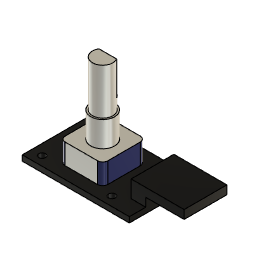
stepper_controller_case v17 (Autodesk Fusion 360 archive; units mm, degrees)
design "UVC_UI_case_KY-040"
Autodesk Fusion 360 part; units mm, degrees
sketch "Sketch1" plane through (0, 0, 0) normal (0, 0, 1) x (1, 0, 0)
  line L0 (4.75, -6.25) -> (-4.75, -6.25)
  line L1 (-6.25, -4.75) -> (-6.25, 4.75)
  line L2 (-4.75, 6.25) -> (4.75, 6.25)
  line L3 (6.25, 4.75) -> (6.25, -4.75)
  line L4 (6.25, -6.25) -> (-6.25, 6.25) construction
  line L5 (-6.25, -6.25) -> (6.25, 6.25) construction
  arc A0 (-4.75, 6.25) -> (-6.25, 4.75) centre (-4.75, 4.75) ccw
  arc A1 (6.25, 4.75) -> (4.75, 6.25) centre (4.75, 4.75) ccw
  arc A2 (4.75, -6.25) -> (6.25, -4.75) centre (4.75, -4.75) ccw
  arc A3 (-6.25, -4.75) -> (-4.75, -6.25) centre (-4.75, -4.75) ccw
  circle A4 centre (0, 0) radius 3.5
  circle A5 centre (0, 0) radius 3
  line L6 (-2.5981, 1.5) -> (2.5981, 1.5)
  line L7 (-6.25, 0) -> (6.25, 0) construction
  line L8 (-13.75, -9.75) -> (17.55, -9.75)
  line L9 (17.55, -9.75) -> (17.55, 9.55)
  line L10 (17.55, 9.55) -> (-13.75, 9.55)
  line L11 (-13.75, 9.55) -> (-13.75, -9.75)
  line L12 (28.75, -4.95) -> (13.25, -4.95)
  line L13 (13.25, -4.95) -> (13.25, 7.55)
  line L14 (13.25, 7.55) -> (28.75, 7.55)
  line L15 (28.75, 7.55) -> (28.75, -4.95)
  circle A6 centre (-10.65, -7.05) radius 1
  circle A7 centre (9.75, -7.05) radius 1
  dimension "d37" = 12.5
  dimension "d38" = 12.5
  dimension "d39" = 1.5
  dimension "d40" = 7
  dimension "d41" = 6
  dimension "d42" = 1.5
  dimension "d43" = 31.3
  dimension "d44" = 19.3
  dimension "d45" = 3.5
  dimension "d46" = 7.5
  dimension "d47" = 15.5
  dimension "d48" = 12.5
  dimension "d49" = 2
  dimension "d50" = 4.3
  dimension "d51" = 2
  dimension "d52" = 3.1
  dimension "d53" = 2.7
  dimension "d54" = 2
  dimension "d55" = 7.8
  dimension "d56" = 2.7
  constraint horizontal L0
  constraint perpendicular L0 L1
  constraint parallel L0 L2
  constraint parallel L1 L3
  constraint coincident L4 A4.centre
  constraint coincident L5 A4.centre
  constraint coincident A4.centre A5.centre
  constraint coincident L4.end L2
  constraint coincident L4.end L1
  constraint tangent L2 A0
  constraint tangent L1 A0
  constraint coincident L5.end L2
  constraint coincident L5.end L3
  constraint tangent L2 A1
  constraint tangent L3 A1
  constraint equal A0 A1
  constraint coincident L4.start L3
  constraint coincident L4.start L0
  constraint tangent L3 A2
  constraint tangent L0 A2
  constraint equal A0 A2
  constraint coincident L5.start L0
  constraint coincident L5.start L1
  constraint tangent L0 A3
  constraint tangent L1 A3
  constraint equal A0 A3
  constraint coincident A5 L6.start
  constraint coincident A5 L6.end
  constraint horizontal L6
  constraint midpoint L1 L7.start
  constraint midpoint L3 L7.end
  constraint horizontal L8
  constraint vertical L9
  constraint horizontal L10
  constraint vertical L11
  constraint horizontal L12
  constraint vertical L13
  constraint horizontal L14
  constraint vertical L15
  measures "d37" distance of L4.end L5.end
  measures "d38" distance of L5.start L4.end
  measures "d39" radius of A0
  measures "d40" diameter of A4
  measures "d41" diameter of A5
  measures "d42" distance of L6 L7
  measures "d43" distance of L8.start L8.end
  measures "d44" distance of L8.start L10.end
  measures "d45" distance of L0 L8
  measures "d46" distance of L1 L11
  measures "d47" distance of L12.start L12.end
  measures "d48" distance of L12.start L14.end
  measures "d49" distance of L10 L14
  measures "d50" distance of L9 L13
  measures "d51" diameter of A6
  measures "d52" distance of L11 A6.centre
  measures "d53" distance of L8 A6.centre
  measures "d54" diameter of A7
  measures "d55" distance of L9 A7.centre
  measures "d56" distance of L8 A7.centre
extrude "Extrude1" add sketch "Sketch1" along normal blind 6 contours L0 L1 L2 L3 A0 A1 A2 A3
extrude "Extrude2" add sketch "Sketch1" along normal blind 13.4 contours A4
extrude "Extrude3" add sketch "Sketch1" along normal blind 17 contours A5 L6 picked at (0.6802, 1.7331)
extrude "Extrude4" add sketch "Sketch1" along normal blind 26.8 contours A5 L6 picked at (-0.5878, 0.191)
extrude "Extrude5" add sketch "Sketch1" 1 faces at (2.0833, -1.5833, 0) against normal blind 1.6 contours L0 L1 L2 L3 A0 A1 A2 A3 | A4 | A5 L6 | A5 L6 | L8 L9 L10 L11 L12 L13 L14 | L9 L12 L13 L14
extrude "Extrude6" add sketch "Sketch1" along normal blind 5 contours L9 L12 L13 L14
extrude "Extrude7" add sketch "Sketch1" along normal blind 2.5 from surface at 2.5 contours L9 L12 L14 L15
move_body "Move1" bodies 1 to x (1, 0, 0) y (0, 1, 0) z (0, 0, 1) at (35, 25, 0)

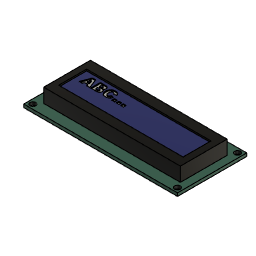
design "UVC_UI_case_LCD_2x16_i2c"
Autodesk Fusion 360 part; units mm, degrees
sketch "display side" plane through (0, 0, 0) normal (0, 0, 1) x (1, 0, 0)
  line L0 (40, 18) -> (-40, 18)
  line L1 (-40, 18) -> (-40, -18)
  line L2 (-40, -18) -> (40, -18)
  line L3 (40, -18) -> (40, 18)
  line L4 (40, 18) -> (-40, -18) construction
  line L5 (-40, 18) -> (40, -18) construction
  line L6 (37.6, -15.65) -> (-37.6, -15.65) construction
  line L7 (-37.6, -15.65) -> (-37.6, 15.65) construction
  line L8 (-37.6, 15.65) -> (37.6, 15.65) construction
  line L9 (37.6, 15.65) -> (37.6, -15.65) construction
  line L10 (37.6, -15.65) -> (-37.6, 15.65) construction
  line L11 (-37.6, -15.65) -> (37.6, 15.65) construction
  circle A0 centre (-37.6, 15.65) radius 1.5
  circle A1 centre (37.6, 15.65) radius 1.5
  circle A2 centre (37.6, -15.65) radius 1.5
  circle A3 centre (-37.6, -15.65) radius 1.5
  line L12 (-35.1, -12.5) -> (36, -12.5)
  line L13 (36, -12.5) -> (36, 11.8)
  line L14 (36, 11.8) -> (-35.1, 11.8)
  line L15 (-35.1, 11.8) -> (-35.1, -12.5)
  line L16 (-32.1, -7.7) -> (32.6, -7.7)
  line L17 (32.6, -7.7) -> (32.6, 6.8)
  line L18 (32.6, 6.8) -> (-32.1, 6.8)
  line L19 (-32.1, 6.8) -> (-32.1, -7.7)
  dimension "d1" = 80
  dimension "d2" = 36
  dimension "d3" = 75.2
  dimension "d4" = 31.3
  dimension "d5" = 3
  dimension "d6" = 3
  dimension "d7" = 3
  dimension "d8" = 3
  dimension "d9" = 71.1
  dimension "d10" = 24.3
  dimension "d11" = 5.5
  dimension "d12" = 4
  dimension "d13" = 14.5
  dimension "d14" = 64.7
  dimension "d15" = 3.4
  dimension "d16" = 4.8
  constraint horizontal L0
  constraint perpendicular L0 L1
  constraint parallel L0 L2
  constraint parallel L1 L3
  constraint coincident L4 origin
  constraint coincident L5 origin
  constraint horizontal L6
  constraint perpendicular L6 L7
  constraint parallel L6 L8
  constraint parallel L7 L9
  constraint coincident L10 origin
  constraint coincident L11 origin
  constraint coincident L7.end L8.start
  constraint coincident L8.end L9.start
  constraint coincident L6.start L9.end
  constraint coincident L6.end L7.start
  constraint horizontal L12
  constraint vertical L13
  constraint horizontal L14
  constraint vertical L15
  constraint horizontal L16
  constraint vertical L17
  constraint horizontal L18
  constraint vertical L19
  measures "d1" distance of L1.end L2.end
  measures "d2" distance of L0.end L1.end
  measures "d3" distance of L7.end L8.end
  measures "d4" distance of L6.end L7.end
  measures "d5" diameter of A0
  measures "d6" diameter of A1
  measures "d7" diameter of A2
  measures "d8" diameter of A3
  measures "d9" distance of L12.start L12.end
  measures "d10" distance of L12.start L14.end
  measures "d11" distance of L2 L12
  measures "d12" distance of L3 L13
  measures "d13" distance of L16.start L18.end
  measures "d14" distance of L17 L19
  measures "d15" distance of L13 L17
  measures "d16" distance of L12 L16
extrude "Extrude1" add sketch "display side" against normal blind 1.6 contours L0 L1 L2 L3 | L12 L13 L14 L15 | L16 L17 L18 L19
extrude "Extrude2" add sketch "display side" along normal blind 7.3 contours L12 L13 L14 L15
extrude "Extrude3" add sketch "display side" along normal blind 6.5 contours L16 L17 L18 L19
sketch "ABC" plane through (0, 0, 6.5) normal (0, 0, 1) x (-1, 0, 0)
  line L0 (32.1, -6.8) -> (32.1, 7.7)
  line L1 (32.1, 7.7) -> (-32.6, 7.7)
  line L2 (-32.6, 7.7) -> (-32.6, -6.8)
  line L3 (-32.6, -6.8) -> (32.1, -6.8)
  line L4 (29.277, -0.034) -> (6.2604, -0.034) construction
  line L5 (6.2604, -0.034) -> (6.2604, -7.034) construction
  line L6 (6.2604, -7.034) -> (29.277, -7.034) construction
  line L7 (29.277, -7.034) -> (29.277, -0.034) construction
  text T0 "ABC..." font "Arial Black" height 7 align ink ink in box 0 x 0 at (29.277, -0.034) x (-1, 0) y (0, -1) spacing 1 kerned height is em
  constraint perpendicular L4 L5
  constraint parallel L4 L6
  constraint parallel L5 L7
extrude "Extrude4" cut sketch "ABC" against normal blind 0.5 text T0
sketch "Bottom" plane through (0, 0, -1.6) normal (0, 0, -1) x (1, 0, 0)
  circle A0 centre (37.6, 15.65) radius 1.5
  circle A1 centre (-37.6, 15.65) radius 1.5
  circle A2 centre (37.6, -15.65) radius 1.5
  circle A3 centre (-37.6, -15.65) radius 1.5
  line L0 (40, -18) -> (40, 18)
  line L1 (40, 18) -> (-40, 18)
  line L2 (-40, 18) -> (-40, -18)
  line L3 (-40, -18) -> (40, -18)
  line L4 (40, 18) -> (-40, 18) construction
  line L5 (-40, 18) -> (-40, -18) construction
  line L6 (-40, -18) -> (40, -18) construction
  line L7 (40, -18) -> (40, 18) construction
  line L8 (-34.5, -17) -> (7.5, -17)
  line L9 (7.5, -17) -> (7.5, 2.5)
  line L10 (7.5, 2.5) -> (-34.5, 2.5)
  line L11 (-34.5, 2.5) -> (-34.5, -17)
  line L12 (-34.5, -1.3) -> (-47.5, -1.3)
  line L13 (-47.5, -1.3) -> (-47.5, -11.3)
  line L14 (-47.5, -11.3) -> (-34.5, -11.3)
  line L15 (-34.5, -11.3) -> (-34.5, -1.3)
  dimension "d25" = 42
  dimension "d26" = 19.5
  dimension "d27" = 1
  dimension "d28" = 5.5
  dimension "d31" = 13
  dimension "d32" = 10
  dimension "d33" = 3.8
  constraint horizontal L8
  constraint vertical L9
  constraint horizontal L10
  constraint vertical L11
  constraint horizontal L12
  constraint vertical L13
  constraint horizontal L14
  constraint vertical L15
  constraint coincident L11 L12.start
  measures "d25" distance of L8.start L8.end
  measures "d26" distance of L8.start L10.end
  measures "d27" distance of L3 L8
  measures "d28" distance of L5 L11
  measures "d31" distance of L12.start L12.end
  measures "d32" distance of L12.start L14.end
  measures "d33" distance of L10 L12
extrude "Extrude5" add sketch "Bottom" along normal blind 8 contours L8 L9 L10 L11 L15
extrude "Extrude6" add sketch "Bottom" along normal blind 3 from surface at 6 contours L2 L12 L13 L14 | L2 L11 L12 L14 L15
equation "d6 = d5"
equation "d7 = d6"
equation "d8 = d7"
named bodies: "display"
